Autodesk Inventor part; units mm, degrees
(part 2 of 3)
  line L420 (576.2805, 16.5874) -> (576.1711, 16.519)
  line L421 (576.1711, 16.519) -> (576.0571, 16.4584)
  line L422 (576.0571, 16.4584) -> (575.9392, 16.4059)
  line L423 (575.9392, 16.4059) -> (575.8179, 16.3617)
  line L424 (575.8179, 16.3617) -> (575.6938, 16.3262)
  line L425 (575.6938, 16.3262) -> (575.5676, 16.2993)
  line L426 (575.5676, 16.2993) -> (575.4398, 16.2814)
  line L427 (575.4398, 16.2814) -> (575.311, 16.2724)
  line L428 (575.311, 16.2724) -> (575.182, 16.2724)
  line L429 (575.182, 16.2724) -> (575.0532, 16.2814)
  line L430 (575.0532, 16.2814) -> (574.9254, 16.2993)
  line L431 (574.9254, 16.2993) -> (574.7992, 16.3262)
  line L432 (574.7992, 16.3262) -> (574.6751, 16.3617)
  line L433 (574.6751, 16.3617) -> (574.5538, 16.4059)
  line L434 (574.5538, 16.4059) -> (574.4359, 16.4584)
  line L435 (574.4359, 16.4584) -> (574.3219, 16.519)
  line L436 (574.3219, 16.519) -> (574.2125, 16.5874)
  line L437 (574.2125, 16.5874) -> (574.1081, 16.6632)
  line L438 (574.1081, 16.6632) -> (574.0092, 16.7462)
  line L439 (574.0092, 16.7462) -> (573.9164, 16.8359)
  line L440 (573.9164, 16.8359) -> (573.83, 16.9318)
  line L441 (573.83, 16.9318) -> (573.7505, 17.0335)
  line L442 (573.7505, 17.0335) -> (573.6784, 17.1405)
  line L443 (573.6784, 17.1405) -> (573.6138, 17.2523)
  line L444 (573.6138, 17.2523) -> (573.5572, 17.3683)
  line L445 (573.5572, 17.3683) -> (573.5089, 17.4879)
  line L446 (573.5089, 17.4879) -> (573.469, 17.6107)
  line L447 (573.469, 17.6107) -> (573.4378, 17.7359)
  line L448 (573.4378, 17.7359) -> (573.4154, 17.863)
  line L449 (573.4154, 17.863) -> (573.4019, 17.9914)
  line L450 (573.4019, 17.9914) -> (573.3974, 18.1204)
  line L451 (573.3974, 18.1204) -> (573.4019, 18.2493)
  line L452 (573.4019, 18.2493) -> (573.4154, 18.3777)
  line L453 (573.4154, 18.3777) -> (573.4378, 18.5048)
  line L454 (573.4378, 18.5048) -> (573.469, 18.63)
  line L455 (573.469, 18.63) -> (573.5089, 18.7528)
  line L456 (573.5089, 18.7528) -> (573.5572, 18.8725)
  line L457 (573.5572, 18.8725) -> (573.6138, 18.9885)
  line L458 (573.6138, 18.9885) -> (573.6784, 19.1002)
  line L459 (573.6784, 19.1002) -> (573.7505, 19.2072)
  line L460 (573.7505, 19.2072) -> (573.83, 19.309)
  line L461 (573.83, 19.309) -> (573.9164, 19.4049)
  line L462 (573.9164, 19.4049) -> (574.0092, 19.4945)
  line L463 (574.0092, 19.4945) -> (574.1081, 19.5775)
  line L464 (574.1081, 19.5775) -> (574.2125, 19.6533)
  line L465 (574.2125, 19.6533) -> (574.3219, 19.7217)
  line L466 (574.3219, 19.7217) -> (574.4359, 19.7823)
  line L467 (574.4359, 19.7823) -> (574.5538, 19.8348)
  line L468 (574.5538, 19.8348) -> (574.6751, 19.879)
  line L469 (574.6751, 19.879) -> (574.7992, 19.9146)
  line L470 (574.7992, 19.9146) -> (574.9254, 19.9414)
  line L471 (574.9254, 19.9414) -> (575.0532, 19.9594)
  line L472 (575.0532, 19.9594) -> (575.182, 19.9684)
  line L473 (575.182, 19.9684) -> (575.311, 19.9684)
  line L474 (575.311, 19.9684) -> (575.4398, 19.9594)
  line L475 (575.4398, 19.9594) -> (575.5676, 19.9414)
  line L476 (575.5676, 19.9414) -> (575.6938, 19.9146)
  line L477 (575.6938, 19.9146) -> (575.8179, 19.879)
  line L478 (575.8179, 19.879) -> (575.9392, 19.8348)
  line L479 (575.9392, 19.8348) -> (576.0571, 19.7823)
  line L480 (576.0571, 19.7823) -> (576.1711, 19.7217)
  line L481 (576.1711, 19.7217) -> (576.2805, 19.6533)
  line L482 (576.2805, 19.6533) -> (576.3849, 19.5775)
  line L483 (576.3849, 19.5775) -> (576.4838, 19.4945)
  line L484 (576.4838, 19.4945) -> (576.5766, 19.4049)
  line L485 (576.5766, 19.4049) -> (576.663, 19.309)
  line L486 (576.663, 19.309) -> (576.7425, 19.2072)
  line L487 (576.7425, 19.2072) -> (576.8146, 19.1002)
  line L488 (576.8146, 19.1002) -> (576.8792, 18.9885)
  line L489 (576.8792, 18.9885) -> (576.9358, 18.8725)
  line L490 (576.9358, 18.8725) -> (576.9841, 18.7528)
  line L491 (576.9841, 18.7528) -> (577.024, 18.63)
  line L492 (577.024, 18.63) -> (577.0552, 18.5048)
  line L493 (577.0552, 18.5048) -> (577.0776, 18.3777)
  line L494 (577.0776, 18.3777) -> (577.0911, 18.2493)
  line L495 (577.0911, 18.2493) -> (577.0956, 18.1204)
  line L496 (314.1597, 166.8545) -> (568.1597, 166.8545)
  line L497 (568.1597, 166.8545) -> (568.1597, 104.8556)
  line L498 (568.1597, 104.8556) -> (314.1597, 104.8556)
  line L499 (314.1597, 104.8556) -> (314.1597, 166.8545)
  line L500 (506.5418, 136.7199) -> (506.585, 137.6267)
  line L501 (506.585, 137.6267) -> (506.7146, 138.5208)
  line L502 (506.7146, 138.5208) -> (506.9254, 139.3996)
  line L503 (506.9254, 139.3996) -> (507.2226, 140.2581)
  line L504 (507.2226, 140.2581) -> (507.601, 141.0785)
  line L505 (507.601, 141.0785) -> (508.0506, 141.8634)
  line L506 (508.0506, 141.8634) -> (508.5764, 142.6025)
  line L507 (508.5764, 142.6025) -> (509.1707, 143.2883)
  line L508 (509.1707, 143.2883) -> (509.8261, 143.9132)
  line L509 (509.8261, 143.9132) -> (510.5398, 144.4694)
  line L510 (510.5398, 144.4694) -> (511.3018, 144.9597)
  line L511 (511.3018, 144.9597) -> (512.1044, 145.3762)
  line L512 (512.1044, 145.3762) -> (512.9452, 145.7115)
  line L513 (512.9452, 145.7115) -> (513.8139, 145.9655)
  line L514 (513.8139, 145.9655) -> (514.6978, 146.1382)
  line L515 (514.6978, 146.1382) -> (515.6046, 146.222)
  line L516 (515.6046, 146.222) -> (516.5113, 146.222)
  line L517 (516.5113, 146.222) -> (517.4105, 146.1382)
  line L518 (517.4105, 146.1382) -> (518.2995, 145.9655)
  line L519 (518.2995, 145.9655) -> (519.1682, 145.7115)
  line L520 (519.1682, 145.7115) -> (520.0115, 145.3762)
  line L521 (520.0115, 145.3762) -> (520.8141, 144.9597)
  line L522 (520.8141, 144.9597) -> (521.5761, 144.4694)
  line L523 (521.5761, 144.4694) -> (522.2873, 143.9132)
  line L524 (522.2873, 143.9132) -> (522.9426, 143.2883)
  line L525 (522.9426, 143.2883) -> (523.5344, 142.6025)
  line L526 (523.5344, 142.6025) -> (524.0602, 141.8634)
  line L527 (524.0602, 141.8634) -> (524.5123, 141.0785)
  line L528 (524.5123, 141.0785) -> (524.8908, 140.2581)
  line L529 (524.8908, 140.2581) -> (525.1854, 139.3996)
  line L530 (525.1854, 139.3996) -> (525.4013, 138.5208)
  line L531 (525.4013, 138.5208) -> (525.5258, 137.6267)
  line L532 (525.5258, 137.6267) -> (525.5715, 136.7199)
  line L533 (525.5715, 136.7199) -> (525.5258, 135.8157)
  line L534 (525.5258, 135.8157) -> (525.4013, 134.919)
  line L535 (525.4013, 134.919) -> (525.1854, 134.0427)
  line L536 (525.1854, 134.0427) -> (524.8908, 133.1842)
  line L537 (524.8908, 133.1842) -> (524.5123, 132.3613)
  line L538 (524.5123, 132.3613) -> (524.0602, 131.5764)
  line L539 (524.0602, 131.5764) -> (523.5344, 130.8373)
  line L540 (523.5344, 130.8373) -> (522.9426, 130.154)
  line L541 (522.9426, 130.154) -> (522.2873, 129.5292)
  line L542 (522.2873, 129.5292) -> (521.5761, 128.9678)
  line L543 (521.5761, 128.9678) -> (520.8141, 128.4827)
  line L544 (520.8141, 128.4827) -> (520.0115, 128.0661)
  line L545 (520.0115, 128.0661) -> (519.1682, 127.7308)
  line L546 (519.1682, 127.7308) -> (518.2995, 127.4718)
  line L547 (518.2995, 127.4718) -> (517.4105, 127.3041)
  line L548 (517.4105, 127.3041) -> (516.5113, 127.2152)
  line L549 (516.5113, 127.2152) -> (515.6046, 127.2152)
  line L550 (515.6046, 127.2152) -> (514.6978, 127.3041)
  line L551 (514.6978, 127.3041) -> (513.8139, 127.4718)
  line L552 (513.8139, 127.4718) -> (512.9452, 127.7308)
  line L553 (512.9452, 127.7308) -> (512.1044, 128.0661)
  line L554 (512.1044, 128.0661) -> (511.3018, 128.4827)
  line L555 (511.3018, 128.4827) -> (510.5398, 128.9678)
  line L556 (510.5398, 128.9678) -> (509.8261, 129.5292)
  line L557 (509.8261, 129.5292) -> (509.1707, 130.154)
  line L558 (509.1707, 130.154) -> (508.5764, 130.8373)
  line L559 (508.5764, 130.8373) -> (508.0506, 131.5764)
  line L560 (508.0506, 131.5764) -> (507.601, 132.3613)
  line L561 (507.601, 132.3613) -> (507.2226, 133.1842)
  line L562 (507.2226, 133.1842) -> (506.9254, 134.0427)
  line L563 (506.9254, 134.0427) -> (506.7146, 134.919)
  line L564 (506.7146, 134.919) -> (506.585, 135.8157)
  line L565 (506.585, 135.8157) -> (506.5418, 136.7199)
  line L566 (401.8837, 136.7199) -> (401.9269, 137.6267)
  line L567 (401.9269, 137.6267) -> (402.0564, 138.5208)
  line L568 (402.0564, 138.5208) -> (402.2647, 139.3996)
  line L569 (402.2647, 139.3996) -> (402.5644, 140.2581)
  line L570 (402.5644, 140.2581) -> (402.9429, 141.0785)
  line L571 (402.9429, 141.0785) -> (403.3924, 141.8634)
  line L572 (403.3924, 141.8634) -> (403.9182, 142.6025)
  line L573 (403.9182, 142.6025) -> (404.5126, 143.2883)
  line L574 (404.5126, 143.2883) -> (405.1679, 143.9132)
  line L575 (405.1679, 143.9132) -> (405.8791, 144.4694)
  line L576 (405.8791, 144.4694) -> (406.6411, 144.9597)
  line L577 (406.6411, 144.9597) -> (407.4463, 145.3762)
  line L578 (407.4463, 145.3762) -> (408.287, 145.7115)
  line L579 (408.287, 145.7115) -> (409.1532, 145.9655)
  line L580 (409.1532, 145.9655) -> (410.0422, 146.1382)
  line L581 (410.0422, 146.1382) -> (410.9464, 146.222)
  line L582 (410.9464, 146.222) -> (411.8481, 146.222)
  line L583 (411.8481, 146.222) -> (412.7523, 146.1382)
  line L584 (412.7523, 146.1382) -> (413.6413, 145.9655)
  line L585 (413.6413, 145.9655) -> (414.51, 145.7115)
  line L586 (414.51, 145.7115) -> (415.3533, 145.3762)
  line L587 (415.3533, 145.3762) -> (416.1534, 144.9597)
  line L588 (416.1534, 144.9597) -> (416.9179, 144.4694)
  line L589 (416.9179, 144.4694) -> (417.6266, 143.9132)
  line L590 (417.6266, 143.9132) -> (418.2845, 143.2883)
  line L591 (418.2845, 143.2883) -> (418.8763, 142.6025)
  line L592 (418.8763, 142.6025) -> (419.4021, 141.8634)
  line L593 (419.4021, 141.8634) -> (419.8542, 141.0785)
  line L594 (419.8542, 141.0785) -> (420.2301, 140.2581)
  line L595 (420.2301, 140.2581) -> (420.5273, 139.3996)
  line L596 (420.5273, 139.3996) -> (420.7381, 138.5208)
  line L597 (420.7381, 138.5208) -> (420.8702, 137.6267)
  line L598 (420.8702, 137.6267) -> (420.9108, 136.7199)
  line L599 (420.9108, 136.7199) -> (420.8702, 135.8157)
  line L600 (420.8702, 135.8157) -> (420.7381, 134.919)
  line L601 (420.7381, 134.919) -> (420.5273, 134.0427)
  line L602 (420.5273, 134.0427) -> (420.2301, 133.1842)
  line L603 (420.2301, 133.1842) -> (419.8542, 132.3613)
  line L604 (419.8542, 132.3613) -> (419.4021, 131.5764)
  line L605 (419.4021, 131.5764) -> (418.8763, 130.8373)
  line L606 (418.8763, 130.8373) -> (418.2845, 130.154)
  line L607 (418.2845, 130.154) -> (417.6266, 129.5292)
  line L608 (417.6266, 129.5292) -> (416.9179, 128.9678)
  line L609 (416.9179, 128.9678) -> (416.1534, 128.4827)
  line L610 (416.1534, 128.4827) -> (415.3533, 128.0661)
  line L611 (415.3533, 128.0661) -> (414.51, 127.7308)
  line L612 (414.51, 127.7308) -> (413.6413, 127.4718)
  line L613 (413.6413, 127.4718) -> (412.7523, 127.3041)
  line L614 (412.7523, 127.3041) -> (411.8481, 127.2152)
  line L615 (411.8481, 127.2152) -> (410.9464, 127.2152)
  line L616 (410.9464, 127.2152) -> (410.0422, 127.3041)
  line L617 (410.0422, 127.3041) -> (409.1532, 127.4718)
  line L618 (409.1532, 127.4718) -> (408.287, 127.7308)
  line L619 (408.287, 127.7308) -> (407.4463, 128.0661)
  line L620 (407.4463, 128.0661) -> (406.6411, 128.4827)
  line L621 (406.6411, 128.4827) -> (405.8791, 128.9678)
  line L622 (405.8791, 128.9678) -> (405.1679, 129.5292)
  line L623 (405.1679, 129.5292) -> (404.5126, 130.154)
  line L624 (404.5126, 130.154) -> (403.9182, 130.8373)
  line L625 (403.9182, 130.8373) -> (403.3924, 131.5764)
  line L626 (403.3924, 131.5764) -> (402.9429, 132.3613)
  line L627 (402.9429, 132.3613) -> (402.5644, 133.1842)
  line L628 (402.5644, 133.1842) -> (402.2647, 134.0427)
  line L629 (402.2647, 134.0427) -> (402.0564, 134.919)
  line L630 (402.0564, 134.919) -> (401.9269, 135.8157)
  line L631 (401.9269, 135.8157) -> (401.8837, 136.7199)
  line L632 (340.0423, 136.7199) -> (340.0829, 137.6267)
  line L633 (340.0829, 137.6267) -> (340.2099, 138.5208)
  line L634 (340.2099, 138.5208) -> (340.4258, 139.3996)
  line L635 (340.4258, 139.3996) -> (340.723, 140.2581)
  line L636 (340.723, 140.2581) -> (341.0964, 141.0785)
  line L637 (341.0964, 141.0785) -> (341.5511, 141.8634)
  line L638 (341.5511, 141.8634) -> (342.0768, 142.6025)
  line L639 (342.0768, 142.6025) -> (342.6687, 143.2883)
  line L640 (342.6687, 143.2883) -> (343.3214, 143.9132)
  line L641 (343.3214, 143.9132) -> (344.0352, 144.4694)
  line L642 (344.0352, 144.4694) -> (344.7972, 144.9597)
  line L643 (344.7972, 144.9597) -> (345.5998, 145.3762)
  line L644 (345.5998, 145.3762) -> (346.4406, 145.7115)
  line L645 (346.4406, 145.7115) -> (347.3118, 145.9655)
  line L646 (347.3118, 145.9655) -> (348.2008, 146.1382)
  line L647 (348.2008, 146.1382) -> (349.0999, 146.222)
  line L648 (349.0999, 146.222) -> (350.0067, 146.222)
  line L649 (350.0067, 146.222) -> (350.9059, 146.1382)
  line L650 (350.9059, 146.1382) -> (351.7949, 145.9655)
  line L651 (351.7949, 145.9655) -> (352.6661, 145.7115)
  line L652 (352.6661, 145.7115) -> (353.5068, 145.3762)
  line L653 (353.5068, 145.3762) -> (354.312, 144.9597)
  line L654 (354.312, 144.9597) -> (355.074, 144.4694)
  line L655 (355.074, 144.4694) -> (355.7852, 143.9132)
  line L656 (355.7852, 143.9132) -> (356.438, 143.2883)
  line L657 (356.438, 143.2883) -> (357.0349, 142.6025)
  line L658 (357.0349, 142.6025) -> (357.5556, 141.8634)
  line L659 (357.5556, 141.8634) -> (358.0128, 141.0785)
  line L660 (358.0128, 141.0785) -> (358.3862, 140.2581)
  line L661 (358.3862, 140.2581) -> (358.6834, 139.3996)
  line L662 (358.6834, 139.3996) -> (358.8942, 138.5208)
  line L663 (358.8942, 138.5208) -> (359.0212, 137.6267)
  line L664 (359.0212, 137.6267) -> (359.0694, 136.7199)
  line L665 (359.0694, 136.7199) -> (359.0212, 135.8157)
  line L666 (359.0212, 135.8157) -> (358.8942, 134.919)
  line L667 (358.8942, 134.919) -> (358.6834, 134.0427)
  line L668 (358.6834, 134.0427) -> (358.3862, 133.1842)
  line L669 (358.3862, 133.1842) -> (358.0128, 132.3613)
  line L670 (358.0128, 132.3613) -> (357.5556, 131.5764)
  line L671 (357.5556, 131.5764) -> (357.0349, 130.8373)
  line L672 (357.0349, 130.8373) -> (356.438, 130.154)
  line L673 (356.438, 130.154) -> (355.7852, 129.5292)
  line L674 (355.7852, 129.5292) -> (355.074, 128.9678)
  line L675 (355.074, 128.9678) -> (354.312, 128.4827)
  line L676 (354.312, 128.4827) -> (353.5068, 128.0661)
  line L677 (353.5068, 128.0661) -> (352.6661, 127.7308)
  line L678 (352.6661, 127.7308) -> (351.7949, 127.4718)
  line L679 (351.7949, 127.4718) -> (350.9059, 127.3041)
  line L680 (350.9059, 127.3041) -> (350.0067, 127.2152)
  line L681 (350.0067, 127.2152) -> (349.0999, 127.2152)
  line L682 (349.0999, 127.2152) -> (348.2008, 127.3041)
  line L683 (348.2008, 127.3041) -> (347.3118, 127.4718)
  line L684 (347.3118, 127.4718) -> (346.4406, 127.7308)
  line L685 (346.4406, 127.7308) -> (345.5998, 128.0661)
  line L686 (345.5998, 128.0661) -> (344.7972, 128.4827)
  line L687 (344.7972, 128.4827) -> (344.0352, 128.9678)
  line L688 (344.0352, 128.9678) -> (343.3214, 129.5292)
  line L689 (343.3214, 129.5292) -> (342.6687, 130.154)
  line L690 (342.6687, 130.154) -> (342.0768, 130.8373)
  line L691 (342.0768, 130.8373) -> (341.5511, 131.5764)
  line L692 (341.5511, 131.5764) -> (341.0964, 132.3613)
  line L693 (341.0964, 132.3613) -> (340.723, 133.1842)
  line L694 (340.723, 133.1842) -> (340.4258, 134.0427)
  line L695 (340.4258, 134.0427) -> (340.2099, 134.919)
  line L696 (340.2099, 134.919) -> (340.0829, 135.8157)
  line L697 (340.0829, 135.8157) -> (340.0423, 136.7199)
  line L698 (319.4988, 163.174) -> (319.4943, 163.045)
  line L699 (319.4943, 163.045) -> (319.4808, 162.9167)
  line L700 (319.4808, 162.9167) -> (319.4584, 162.7895)
  line L701 (319.4584, 162.7895) -> (319.4271, 162.6643)
  line L702 (319.4271, 162.6643) -> (319.3873, 162.5416)
  line L703 (319.3873, 162.5416) -> (319.3389, 162.4219)
  line L704 (319.3389, 162.4219) -> (319.2823, 162.3059)
  line L705 (319.2823, 162.3059) -> (319.2178, 162.1941)
  line L706 (319.2178, 162.1941) -> (319.1456, 162.0871)
  line L707 (319.1456, 162.0871) -> (319.0662, 161.9854)
  line L708 (319.0662, 161.9854) -> (318.9798, 161.8895)
  line L709 (318.9798, 161.8895) -> (318.887, 161.7998)
  line L710 (318.887, 161.7998) -> (318.7881, 161.7169)
  line L711 (318.7881, 161.7169) -> (318.6837, 161.641)
  line L712 (318.6837, 161.641) -> (318.5742, 161.5726)
  line L713 (318.5742, 161.5726) -> (318.4603, 161.512)
  line L714 (318.4603, 161.512) -> (318.3424, 161.4595)
  line L715 (318.3424, 161.4595) -> (318.2211, 161.4154)
  line L716 (318.2211, 161.4154) -> (318.097, 161.3798)
  line L717 (318.097, 161.3798) -> (317.9708, 161.353)
  line L718 (317.9708, 161.353) -> (317.8429, 161.335)
  line L719 (317.8429, 161.335) -> (317.7142, 161.326)
  line L720 (317.7142, 161.326) -> (317.5851, 161.326)
  line L721 (317.5851, 161.326) -> (317.4564, 161.335)
  line L722 (317.4564, 161.335) -> (317.3286, 161.353)
  line L723 (317.3286, 161.353) -> (317.2023, 161.3798)
  line L724 (317.2023, 161.3798) -> (317.0783, 161.4154)
  line L725 (317.0783, 161.4154) -> (316.957, 161.4595)
  line L726 (316.957, 161.4595) -> (316.8391, 161.512)
  line L727 (316.8391, 161.512) -> (316.7251, 161.5726)
  line L728 (316.7251, 161.5726) -> (316.6156, 161.641)
  line L729 (316.6156, 161.641) -> (316.5112, 161.7169)
  line L730 (316.5112, 161.7169) -> (316.4124, 161.7998)
  line L731 (316.4124, 161.7998) -> (316.3195, 161.8895)
  line L732 (316.3195, 161.8895) -> (316.2332, 161.9854)
  line L733 (316.2332, 161.9854) -> (316.1537, 162.0871)
  line L734 (316.1537, 162.0871) -> (316.0815, 162.1941)
  line L735 (316.0815, 162.1941) -> (316.017, 162.3059)
  line L736 (316.017, 162.3059) -> (315.9604, 162.4219)
  line L737 (315.9604, 162.4219) -> (315.9121, 162.5416)
  line L738 (315.9121, 162.5416) -> (315.8722, 162.6643)
  line L739 (315.8722, 162.6643) -> (315.8409, 162.7895)
  line L740 (315.8409, 162.7895) -> (315.8185, 162.9167)
  line L741 (315.8185, 162.9167) -> (315.805, 163.045)
  line L742 (315.805, 163.045) -> (315.8005, 163.174)
  line L743 (315.8005, 163.174) -> (315.805, 163.303)
  line L744 (315.805, 163.303) -> (315.8185, 163.4313)
  line L745 (315.8185, 163.4313) -> (315.8409, 163.5585)
  line L746 (315.8409, 163.5585) -> (315.8722, 163.6837)
  line L747 (315.8722, 163.6837) -> (315.9121, 163.8064)
  line L748 (315.9121, 163.8064) -> (315.9604, 163.9261)
  line L749 (315.9604, 163.9261) -> (316.017, 164.0421)
  line L750 (316.017, 164.0421) -> (316.0815, 164.1539)
  line L751 (316.0815, 164.1539) -> (316.1537, 164.2609)
  line L752 (316.1537, 164.2609) -> (316.2332, 164.3626)
  line L753 (316.2332, 164.3626) -> (316.3195, 164.4585)
  line L754 (316.3195, 164.4585) -> (316.4124, 164.5482)
  line L755 (316.4124, 164.5482) -> (316.5112, 164.6311)
  line L756 (316.5112, 164.6311) -> (316.6156, 164.707)
  line L757 (316.6156, 164.707) -> (316.7251, 164.7754)
  line L758 (316.7251, 164.7754) -> (316.8391, 164.836)
  line L759 (316.8391, 164.836) -> (316.957, 164.8885)
  line L760 (316.957, 164.8885) -> (317.0783, 164.9326)
  line L761 (317.0783, 164.9326) -> (317.2023, 164.9682)
  line L762 (317.2023, 164.9682) -> (317.3286, 164.995)
  line L763 (317.3286, 164.995) -> (317.4564, 165.013)
  line L764 (317.4564, 165.013) -> (317.5851, 165.022)
  line L765 (317.5851, 165.022) -> (317.7142, 165.022)
  line L766 (317.7142, 165.022) -> (317.8429, 165.013)
  line L767 (317.8429, 165.013) -> (317.9708, 164.995)
  line L768 (317.9708, 164.995) -> (318.097, 164.9682)
  line L769 (318.097, 164.9682) -> (318.2211, 164.9326)
  line L770 (318.2211, 164.9326) -> (318.3424, 164.8885)
  line L771 (318.3424, 164.8885) -> (318.4603, 164.836)
  line L772 (318.4603, 164.836) -> (318.5742, 164.7754)
  line L773 (318.5742, 164.7754) -> (318.6837, 164.707)
  line L774 (318.6837, 164.707) -> (318.7881, 164.6311)
  line L775 (318.7881, 164.6311) -> (318.887, 164.5482)
  line L776 (318.887, 164.5482) -> (318.9798, 164.4585)
  line L777 (318.9798, 164.4585) -> (319.0662, 164.3626)
  line L778 (319.0662, 164.3626) -> (319.1456, 164.2609)
  line L779 (319.1456, 164.2609) -> (319.2178, 164.1539)
  line L780 (319.2178, 164.1539) -> (319.2823, 164.0421)
  line L781 (319.2823, 164.0421) -> (319.3389, 163.9261)
  line L782 (319.3389, 163.9261) -> (319.3873, 163.8064)
  line L783 (319.3873, 163.8064) -> (319.4271, 163.6837)
  line L784 (319.4271, 163.6837) -> (319.4584, 163.5585)
  line L785 (319.4584, 163.5585) -> (319.4808, 163.4313)
  line L786 (319.4808, 163.4313) -> (319.4943, 163.303)
  line L787 (319.4943, 163.303) -> (319.4988, 163.174)
  line L788 (319.4988, 108.9831) -> (319.4943, 108.8541)
  line L789 (319.4943, 108.8541) -> (319.4808, 108.7258)
  line L790 (319.4808, 108.7258) -> (319.4584, 108.5986)
  line L791 (319.4584, 108.5986) -> (319.4271, 108.4734)
  line L792 (319.4271, 108.4734) -> (319.3873, 108.3507)
  line L793 (319.3873, 108.3507) -> (319.3389, 108.231)
  line L794 (319.3389, 108.231) -> (319.2823, 108.115)
  line L795 (319.2823, 108.115) -> (319.2178, 108.0032)
  line L796 (319.2178, 108.0032) -> (319.1456, 107.8962)
  line L797 (319.1456, 107.8962) -> (319.0662, 107.7945)
  line L798 (319.0662, 107.7945) -> (318.9798, 107.6986)
  line L799 (318.9798, 107.6986) -> (318.887, 107.6089)
  line L800 (318.887, 107.6089) -> (318.7881, 107.526)
  line L801 (318.7881, 107.526) -> (318.6837, 107.4501)
  line L802 (318.6837, 107.4501) -> (318.5742, 107.3817)
  line L803 (318.5742, 107.3817) -> (318.4603, 107.3211)
  line L804 (318.4603, 107.3211) -> (318.3424, 107.2686)
  line L805 (318.3424, 107.2686) -> (318.2211, 107.2245)
  line L806 (318.2211, 107.2245) -> (318.097, 107.1889)
  line L807 (318.097, 107.1889) -> (317.9708, 107.1621)
  line L808 (317.9708, 107.1621) -> (317.8429, 107.1441)
  line L809 (317.8429, 107.1441) -> (317.7142, 107.1351)
  line L810 (317.7142, 107.1351) -> (317.5851, 107.1351)
  line L811 (317.5851, 107.1351) -> (317.4564, 107.1441)
  line L812 (317.4564, 107.1441) -> (317.3286, 107.1621)
  line L813 (317.3286, 107.1621) -> (317.2023, 107.1889)
  line L814 (317.2023, 107.1889) -> (317.0783, 107.2245)
  line L815 (317.0783, 107.2245) -> (316.957, 107.2686)
  line L816 (316.957, 107.2686) -> (316.8391, 107.3211)
  line L817 (316.8391, 107.3211) -> (316.7251, 107.3817)
  line L818 (316.7251, 107.3817) -> (316.6156, 107.4501)
  line L819 (316.6156, 107.4501) -> (316.5112, 107.526)
  line L820 (316.5112, 107.526) -> (316.4124, 107.6089)
  line L821 (316.4124, 107.6089) -> (316.3195, 107.6986)
  line L822 (316.3195, 107.6986) -> (316.2332, 107.7945)
  line L823 (316.2332, 107.7945) -> (316.1537, 107.8962)
  line L824 (316.1537, 107.8962) -> (316.0815, 108.0032)
  line L825 (316.0815, 108.0032) -> (316.017, 108.115)
  line L826 (316.017, 108.115) -> (315.9604, 108.231)
  line L827 (315.9604, 108.231) -> (315.9121, 108.3507)
  line L828 (315.9121, 108.3507) -> (315.8722, 108.4734)
  line L829 (315.8722, 108.4734) -> (315.8409, 108.5986)
  line L830 (315.8409, 108.5986) -> (315.8185, 108.7258)
  line L831 (315.8185, 108.7258) -> (315.805, 108.8541)
  line L832 (315.805, 108.8541) -> (315.8005, 108.9831)
  line L833 (315.8005, 108.9831) -> (315.805, 109.1121)
  line L834 (315.805, 109.1121) -> (315.8185, 109.2404)
  line L835 (315.8185, 109.2404) -> (315.8409, 109.3676)
  line L836 (315.8409, 109.3676) -> (315.8722, 109.4928)
  line L837 (315.8722, 109.4928) -> (315.9121, 109.6155)
  line L838 (315.9121, 109.6155) -> (315.9604, 109.7352)
  line L839 (315.9604, 109.7352) -> (316.017, 109.8512)
  line L840 (316.017, 109.8512) -> (316.0815, 109.963)
  line L841 (316.0815, 109.963) -> (316.1537, 110.07)
  line L842 (316.1537, 110.07) -> (316.2332, 110.1717)
  line L843 (316.2332, 110.1717) -> (316.3195, 110.2676)
  line L844 (316.3195, 110.2676) -> (316.4124, 110.3573)
  line L845 (316.4124, 110.3573) -> (316.5112, 110.4402)
  line L846 (316.5112, 110.4402) -> (316.6156, 110.5161)
  line L847 (316.6156, 110.5161) -> (316.7251, 110.5845)
  line L848 (316.7251, 110.5845) -> (316.8391, 110.6451)
  line L849 (316.8391, 110.6451) -> (316.957, 110.6976)
  line L850 (316.957, 110.6976) -> (317.0783, 110.7417)
  line L851 (317.0783, 110.7417) -> (317.2023, 110.7773)
  line L852 (317.2023, 110.7773) -> (317.3286, 110.8041)
  line L853 (317.3286, 110.8041) -> (317.4564, 110.8221)
  line L854 (317.4564, 110.8221) -> (317.5851, 110.8311)
  line L855 (317.5851, 110.8311) -> (317.7142, 110.8311)
  line L856 (317.7142, 110.8311) -> (317.8429, 110.8221)
  line L857 (317.8429, 110.8221) -> (317.9708, 110.8041)
  line L858 (317.9708, 110.8041) -> (318.097, 110.7773)
  line L859 (318.097, 110.7773) -> (318.2211, 110.7417)
  line L860 (318.2211, 110.7417) -> (318.3424, 110.6976)
  line L861 (318.3424, 110.6976) -> (318.4603, 110.6451)
  line L862 (318.4603, 110.6451) -> (318.5742, 110.5845)
  line L863 (318.5742, 110.5845) -> (318.6837, 110.5161)
  line L864 (318.6837, 110.5161) -> (318.7881, 110.4402)
  line L865 (318.7881, 110.4402) -> (318.887, 110.3573)
  line L866 (318.887, 110.3573) -> (318.9798, 110.2676)
  line L867 (318.9798, 110.2676) -> (319.0662, 110.1717)
  line L868 (319.0662, 110.1717) -> (319.1456, 110.07)
  line L869 (319.1456, 110.07) -> (319.2178, 109.963)
  line L870 (319.2178, 109.963) -> (319.2823, 109.8512)
  line L871 (319.2823, 109.8512) -> (319.3389, 109.7352)
  line L872 (319.3389, 109.7352) -> (319.3873, 109.6155)
  line L873 (319.3873, 109.6155) -> (319.4271, 109.4928)
  line L874 (319.4271, 109.4928) -> (319.4584, 109.3676)
  line L875 (319.4584, 109.3676) -> (319.4808, 109.2404)
  line L876 (319.4808, 109.2404) -> (319.4943, 109.1121)
  line L877 (319.4943, 109.1121) -> (319.4988, 108.9831)
  line L878 (565.8483, 108.9831) -> (565.8438, 108.8541)
  line L879 (565.8438, 108.8541) -> (565.8303, 108.7258)
  line L880 (565.8303, 108.7258) -> (565.8079, 108.5986)
  line L881 (565.8079, 108.5986) -> (565.7767, 108.4734)
  line L882 (565.7767, 108.4734) -> (565.7368, 108.3507)
  line L883 (565.7368, 108.3507) -> (565.6884, 108.231)
  line L884 (565.6884, 108.231) -> (565.6319, 108.115)
  line L885 (565.6319, 108.115) -> (565.5673, 108.0032)
  line L886 (565.5673, 108.0032) -> (565.4951, 107.8962)
  line L887 (565.4951, 107.8962) -> (565.4157, 107.7945)
  line L888 (565.4157, 107.7945) -> (565.3293, 107.6986)
  line L889 (565.3293, 107.6986) -> (565.2365, 107.6089)
  line L890 (565.2365, 107.6089) -> (565.1376, 107.526)
  line L891 (565.1376, 107.526) -> (565.0332, 107.4501)
  line L892 (565.0332, 107.4501) -> (564.9237, 107.3817)
  line L893 (564.9237, 107.3817) -> (564.8098, 107.3211)
  line L894 (564.8098, 107.3211) -> (564.6919, 107.2686)
  line L895 (564.6919, 107.2686) -> (564.5706, 107.2245)
  line L896 (564.5706, 107.2245) -> (564.4465, 107.1889)
  line L897 (564.4465, 107.1889) -> (564.3203, 107.1621)
  line L898 (564.3203, 107.1621) -> (564.1925, 107.1441)
  line L899 (564.1925, 107.1441) -> (564.0637, 107.1351)
  line L900 (564.0637, 107.1351) -> (563.9346, 107.1351)
  line L901 (563.9346, 107.1351) -> (563.8059, 107.1441)
  line L902 (563.8059, 107.1441) -> (563.6781, 107.1621)
  line L903 (563.6781, 107.1621) -> (563.5518, 107.1889)
  line L904 (563.5518, 107.1889) -> (563.4278, 107.2245)
  line L905 (563.4278, 107.2245) -> (563.3065, 107.2686)
  line L906 (563.3065, 107.2686) -> (563.1886, 107.3211)
  line L907 (563.1886, 107.3211) -> (563.0746, 107.3817)
  line L908 (563.0746, 107.3817) -> (562.9652, 107.4501)
  line L909 (562.9652, 107.4501) -> (562.8607, 107.526)
  line L910 (562.8607, 107.526) -> (562.7619, 107.6089)
  line L911 (562.7619, 107.6089) -> (562.669, 107.6986)
  line L912 (562.669, 107.6986) -> (562.5827, 107.7945)
  line L913 (562.5827, 107.7945) -> (562.5032, 107.8962)
  line L914 (562.5032, 107.8962) -> (562.431, 108.0032)
  line L915 (562.431, 108.0032) -> (562.3665, 108.115)
  line L916 (562.3665, 108.115) -> (562.3099, 108.231)
  line L917 (562.3099, 108.231) -> (562.2616, 108.3507)
  line L918 (562.2616, 108.3507) -> (562.2217, 108.4734)
  line L919 (562.2217, 108.4734) -> (562.1905, 108.5986)
  line L920 (562.1905, 108.5986) -> (562.1681, 108.7258)
  line L921 (562.1681, 108.7258) -> (562.1546, 108.8541)
  line L922 (562.1546, 108.8541) -> (562.1501, 108.9831)
  line L923 (562.1501, 108.9831) -> (562.1546, 109.1121)
  line L924 (562.1546, 109.1121) -> (562.1681, 109.2404)
  line L925 (562.1681, 109.2404) -> (562.1905, 109.3676)
  line L926 (562.1905, 109.3676) -> (562.2217, 109.4928)
  line L927 (562.2217, 109.4928) -> (562.2616, 109.6155)
  line L928 (562.2616, 109.6155) -> (562.3099, 109.7352)
  line L929 (562.3099, 109.7352) -> (562.3665, 109.8512)
  line L930 (562.3665, 109.8512) -> (562.431, 109.963)
  line L931 (562.431, 109.963) -> (562.5032, 110.07)
  line L932 (562.5032, 110.07) -> (562.5827, 110.1717)
  line L933 (562.5827, 110.1717) -> (562.669, 110.2676)
  line L934 (562.669, 110.2676) -> (562.7619, 110.3573)
  line L935 (562.7619, 110.3573) -> (562.8607, 110.4402)
  line L936 (562.8607, 110.4402) -> (562.9652, 110.5161)
  line L937 (562.9652, 110.5161) -> (563.0746, 110.5845)
  line L938 (563.0746, 110.5845) -> (563.1886, 110.6451)
  line L939 (563.1886, 110.6451) -> (563.3065, 110.6976)
  line L940 (563.3065, 110.6976) -> (563.4278, 110.7417)
  line L941 (563.4278, 110.7417) -> (563.5518, 110.7773)
  line L942 (563.5518, 110.7773) -> (563.6781, 110.8041)
  line L943 (563.6781, 110.8041) -> (563.8059, 110.8221)
  line L944 (563.8059, 110.8221) -> (563.9346, 110.8311)
  line L945 (563.9346, 110.8311) -> (564.0637, 110.8311)
  line L946 (564.0637, 110.8311) -> (564.1925, 110.8221)
  line L947 (564.1925, 110.8221) -> (564.3203, 110.8041)
  line L948 (564.3203, 110.8041) -> (564.4465, 110.7773)
  line L949 (564.4465, 110.7773) -> (564.5706, 110.7417)
  line L950 (564.5706, 110.7417) -> (564.6919, 110.6976)
  line L951 (564.6919, 110.6976) -> (564.8098, 110.6451)
  line L952 (564.8098, 110.6451) -> (564.9237, 110.5845)
  line L953 (564.9237, 110.5845) -> (565.0332, 110.5161)
  line L954 (565.0332, 110.5161) -> (565.1376, 110.4402)
  line L955 (565.1376, 110.4402) -> (565.2365, 110.3573)
  line L956 (565.2365, 110.3573) -> (565.3293, 110.2676)
  line L957 (565.3293, 110.2676) -> (565.4157, 110.1717)
  line L958 (565.4157, 110.1717) -> (565.4951, 110.07)
  line L959 (565.4951, 110.07) -> (565.5673, 109.963)
  line L960 (565.5673, 109.963) -> (565.6319, 109.8512)
  line L961 (565.6319, 109.8512) -> (565.6884, 109.7352)
  line L962 (565.6884, 109.7352) -> (565.7368, 109.6155)
  line L963 (565.7368, 109.6155) -> (565.7767, 109.4928)
  line L964 (565.7767, 109.4928) -> (565.8079, 109.3676)
  line L965 (565.8079, 109.3676) -> (565.8303, 109.2404)
  line L966 (565.8303, 109.2404) -> (565.8438, 109.1121)
  line L967 (565.8438, 109.1121) -> (565.8483, 108.9831)
  line L968 (565.8483, 163.174) -> (565.8438, 163.045)
  line L969 (565.8438, 163.045) -> (565.8303, 162.9167)
  line L970 (565.8303, 162.9167) -> (565.8079, 162.7895)
  line L971 (565.8079, 162.7895) -> (565.7767, 162.6643)
  line L972 (565.7767, 162.6643) -> (565.7368, 162.5416)
  line L973 (565.7368, 162.5416) -> (565.6884, 162.4219)
  line L974 (565.6884, 162.4219) -> (565.6319, 162.3059)
  line L975 (565.6319, 162.3059) -> (565.5673, 162.1941)
  line L976 (565.5673, 162.1941) -> (565.4951, 162.0871)
  line L977 (565.4951, 162.0871) -> (565.4157, 161.9854)
  line L978 (565.4157, 161.9854) -> (565.3293, 161.8895)
  line L979 (565.3293, 161.8895) -> (565.2365, 161.7998)
  line L980 (565.2365, 161.7998) -> (565.1376, 161.7169)
  line L981 (565.1376, 161.7169) -> (565.0332, 161.641)
  line L982 (565.0332, 161.641) -> (564.9237, 161.5726)
  line L983 (564.9237, 161.5726) -> (564.8098, 161.512)
  line L984 (564.8098, 161.512) -> (564.6919, 161.4595)
  line L985 (564.6919, 161.4595) -> (564.5706, 161.4154)
  line L986 (564.5706, 161.4154) -> (564.4465, 161.3798)
  line L987 (564.4465, 161.3798) -> (564.3203, 161.353)
  line L988 (564.3203, 161.353) -> (564.1925, 161.335)
  line L989 (564.1925, 161.335) -> (564.0637, 161.326)
  line L990 (564.0637, 161.326) -> (563.9346, 161.326)
  line L991 (563.9346, 161.326) -> (563.8059, 161.335)
  line L992 (563.8059, 161.335) -> (563.6781, 161.353)
  line L993 (563.6781, 161.353) -> (563.5518, 161.3798)
  line L994 (563.5518, 161.3798) -> (563.4278, 161.4154)
  line L995 (563.4278, 161.4154) -> (563.3065, 161.4595)
  line L996 (563.3065, 161.4595) -> (563.1886, 161.512)
  line L997 (563.1886, 161.512) -> (563.0746, 161.5726)
  line L998 (563.0746, 161.5726) -> (562.9652, 161.641)
  line L999 (562.9652, 161.641) -> (562.8607, 161.7169)
  line L1000 (562.8607, 161.7169) -> (562.7619, 161.7998)
  line L1001 (562.7619, 161.7998) -> (562.669, 161.8895)
  line L1002 (562.669, 161.8895) -> (562.5827, 161.9854)
  line L1003 (562.5827, 161.9854) -> (562.5032, 162.0871)
  line L1004 (562.5032, 162.0871) -> (562.431, 162.1941)
  line L1005 (562.431, 162.1941) -> (562.3665, 162.3059)
  line L1006 (562.3665, 162.3059) -> (562.3099, 162.4219)
  line L1007 (562.3099, 162.4219) -> (562.2616, 162.5416)
  line L1008 (562.2616, 162.5416) -> (562.2217, 162.6643)
  line L1009 (562.2217, 162.6643) -> (562.1905, 162.7895)
  line L1010 (562.1905, 162.7895) -> (562.1681, 162.9167)
  line L1011 (562.1681, 162.9167) -> (562.1546, 163.045)
  line L1012 (562.1546, 163.045) -> (562.1501, 163.174)
  line L1013 (562.1501, 163.174) -> (562.1546, 163.303)
  line L1014 (562.1546, 163.303) -> (562.1681, 163.4313)
  line L1015 (562.1681, 163.4313) -> (562.1905, 163.5585)
  line L1016 (562.1905, 163.5585) -> (562.2217, 163.6837)
  line L1017 (562.2217, 163.6837) -> (562.2616, 163.8064)
  line L1018 (562.2616, 163.8064) -> (562.3099, 163.9261)
  line L1019 (562.3099, 163.9261) -> (562.3665, 164.0421)
  line L1020 (562.3665, 164.0421) -> (562.431, 164.1539)
  line L1021 (562.431, 164.1539) -> (562.5032, 164.2609)
  line L1022 (562.5032, 164.2609) -> (562.5827, 164.3626)
  line L1023 (562.5827, 164.3626) -> (562.669, 164.4585)
  line L1024 (562.669, 164.4585) -> (562.7619, 164.5482)
  line L1025 (562.7619, 164.5482) -> (562.8607, 164.6311)
  line L1026 (562.8607, 164.6311) -> (562.9652, 164.707)
  line L1027 (562.9652, 164.707) -> (563.0746, 164.7754)
  line L1028 (563.0746, 164.7754) -> (563.1886, 164.836)
  line L1029 (563.1886, 164.836) -> (563.3065, 164.8885)
  line L1030 (563.3065, 164.8885) -> (563.4278, 164.9326)
  line L1031 (563.4278, 164.9326) -> (563.5518, 164.9682)
  line L1032 (563.5518, 164.9682) -> (563.6781, 164.995)
  line L1033 (563.6781, 164.995) -> (563.8059, 165.013)
  line L1034 (563.8059, 165.013) -> (563.9346, 165.022)
  line L1035 (563.9346, 165.022) -> (564.0637, 165.022)
  line L1036 (564.0637, 165.022) -> (564.1925, 165.013)
  line L1037 (564.1925, 165.013) -> (564.3203, 164.995)
  line L1038 (564.3203, 164.995) -> (564.4465, 164.9682)
  line L1039 (564.4465, 164.9682) -> (564.5706, 164.9326)
  line L1040 (564.5706, 164.9326) -> (564.6919, 164.8885)
  line L1041 (564.6919, 164.8885) -> (564.8098, 164.836)
  line L1042 (564.8098, 164.836) -> (564.9237, 164.7754)
  line L1043 (564.9237, 164.7754) -> (565.0332, 164.707)
  line L1044 (565.0332, 164.707) -> (565.1376, 164.6311)
  line L1045 (565.1376, 164.6311) -> (565.2365, 164.5482)
  line L1046 (565.2365, 164.5482) -> (565.3293, 164.4585)
  line L1047 (565.3293, 164.4585) -> (565.4157, 164.3626)
  line L1048 (565.4157, 164.3626) -> (565.4951, 164.2609)
  line L1049 (565.4951, 164.2609) -> (565.5673, 164.1539)
  line L1050 (565.5673, 164.1539) -> (565.6319, 164.0421)
  line L1051 (565.6319, 164.0421) -> (565.6884, 163.9261)
  line L1052 (565.6884, 163.9261) -> (565.7368, 163.8064)
  line L1053 (565.7368, 163.8064) -> (565.7767, 163.6837)
  line L1054 (565.7767, 163.6837) -> (565.8079, 163.5585)
  line L1055 (565.8079, 163.5585) -> (565.8303, 163.4313)
  line L1056 (565.8303, 163.4313) -> (565.8438, 163.303)
  line L1057 (565.8438, 163.303) -> (565.8483, 163.174)
  line L1058 (419.7983, 121.6831) -> (419.7938, 121.5541)
  line L1059 (419.7938, 121.5541) -> (419.7803, 121.4258)
  line L1060 (419.7803, 121.4258) -> (419.7579, 121.2986)
  line L1061 (419.7579, 121.2986) -> (419.7267, 121.1734)
  line L1062 (419.7267, 121.1734) -> (419.6868, 121.0507)
  line L1063 (419.6868, 121.0507) -> (419.6384, 120.931)
  line L1064 (419.6384, 120.931) -> (419.5819, 120.815)
  line L1065 (419.5819, 120.815) -> (419.5173, 120.7032)
  line L1066 (419.5173, 120.7032) -> (419.4451, 120.5962)
  line L1067 (419.4451, 120.5962) -> (419.3657, 120.4945)
  line L1068 (419.3657, 120.4945) -> (419.2793, 120.3986)
  line L1069 (419.2793, 120.3986) -> (419.1865, 120.3089)
  line L1070 (419.1865, 120.3089) -> (419.0876, 120.226)
  line L1071 (419.0876, 120.226) -> (418.9832, 120.1501)
  line L1072 (418.9832, 120.1501) -> (418.8737, 120.0817)
  line L1073 (418.8737, 120.0817) -> (418.7598, 120.0211)
  line L1074 (418.7598, 120.0211) -> (418.6419, 119.9686)
  line L1075 (418.6419, 119.9686) -> (418.5206, 119.9245)
  line L1076 (418.5206, 119.9245) -> (418.3965, 119.8889)
  line L1077 (418.3965, 119.8889) -> (418.2703, 119.8621)
  line L1078 (418.2703, 119.8621) -> (418.1425, 119.8441)
  line L1079 (418.1425, 119.8441) -> (418.0137, 119.8351)
  line L1080 (418.0137, 119.8351) -> (417.8846, 119.8351)
  line L1081 (417.8846, 119.8351) -> (417.7559, 119.8441)
  line L1082 (417.7559, 119.8441) -> (417.6281, 119.8621)
  line L1083 (417.6281, 119.8621) -> (417.5018, 119.8889)
  line L1084 (417.5018, 119.8889) -> (417.3778, 119.9245)
  line L1085 (417.3778, 119.9245) -> (417.2565, 119.9686)
  line L1086 (417.2565, 119.9686) -> (417.1386, 120.0211)
  line L1087 (417.1386, 120.0211) -> (417.0246, 120.0817)
  line L1088 (417.0246, 120.0817) -> (416.9152, 120.1501)
  line L1089 (416.9152, 120.1501) -> (416.8107, 120.226)
  line L1090 (416.8107, 120.226) -> (416.7119, 120.3089)
  line L1091 (416.7119, 120.3089) -> (416.619, 120.3986)
  line L1092 (416.619, 120.3986) -> (416.5327, 120.4945)
  line L1093 (416.5327, 120.4945) -> (416.4532, 120.5962)
  line L1094 (416.4532, 120.5962) -> (416.381, 120.7032)
  line L1095 (416.381, 120.7032) -> (416.3165, 120.815)
  line L1096 (416.3165, 120.815) -> (416.2599, 120.931)
  line L1097 (416.2599, 120.931) -> (416.2116, 121.0507)
  line L1098 (416.2116, 121.0507) -> (416.1717, 121.1734)
  line L1099 (416.1717, 121.1734) -> (416.1405, 121.2986)
  line L1100 (416.1405, 121.2986) -> (416.1181, 121.4258)
  line L1101 (416.1181, 121.4258) -> (416.1046, 121.5541)
  line L1102 (416.1046, 121.5541) -> (416.1001, 121.6831)
  line L1103 (416.1001, 121.6831) -> (416.1046, 121.8121)
  line L1104 (416.1046, 121.8121) -> (416.1181, 121.9404)
  line L1105 (416.1181, 121.9404) -> (416.1405, 122.0676)
  line L1106 (416.1405, 122.0676) -> (416.1717, 122.1928)
  line L1107 (416.1717, 122.1928) -> (416.2116, 122.3155)
  line L1108 (416.2116, 122.3155) -> (416.2599, 122.4352)
  line L1109 (416.2599, 122.4352) -> (416.3165, 122.5512)
  line L1110 (416.3165, 122.5512) -> (416.381, 122.663)
  line L1111 (416.381, 122.663) -> (416.4532, 122.77)
  line L1112 (416.4532, 122.77) -> (416.5327, 122.8717)
  line L1113 (416.5327, 122.8717) -> (416.619, 122.9676)
  line L1114 (416.619, 122.9676) -> (416.7119, 123.0573)
  line L1115 (416.7119, 123.0573) -> (416.8107, 123.1402)
  line L1116 (416.8107, 123.1402) -> (416.9152, 123.2161)
  line L1117 (416.9152, 123.2161) -> (417.0246, 123.2845)
  line L1118 (417.0246, 123.2845) -> (417.1386, 123.3451)
  line L1119 (417.1386, 123.3451) -> (417.2565, 123.3976)
  line L1120 (417.2565, 123.3976) -> (417.3778, 123.4417)
  line L1121 (417.3778, 123.4417) -> (417.5018, 123.4773)
  line L1122 (417.5018, 123.4773) -> (417.6281, 123.5041)
  line L1123 (417.6281, 123.5041) -> (417.7559, 123.5221)
  line L1124 (417.7559, 123.5221) -> (417.8846, 123.5311)
  line L1125 (417.8846, 123.5311) -> (418.0137, 123.5311)
  line L1126 (418.0137, 123.5311) -> (418.1425, 123.5221)
  line L1127 (418.1425, 123.5221) -> (418.2703, 123.5041)
  line L1128 (418.2703, 123.5041) -> (418.3965, 123.4773)
  line L1129 (418.3965, 123.4773) -> (418.5206, 123.4417)
  line L1130 (418.5206, 123.4417) -> (418.6419, 123.3976)
  line L1131 (418.6419, 123.3976) -> (418.7598, 123.3451)
  line L1132 (418.7598, 123.3451) -> (418.8737, 123.2845)
  line L1133 (418.8737, 123.2845) -> (418.9832, 123.2161)
  line L1134 (418.9832, 123.2161) -> (419.0876, 123.1402)
  line L1135 (419.0876, 123.1402) -> (419.1865, 123.0573)
  line L1136 (419.1865, 123.0573) -> (419.2793, 122.9676)
  line L1137 (419.2793, 122.9676) -> (419.3657, 122.8717)
  line L1138 (419.3657, 122.8717) -> (419.4451, 122.77)
  line L1139 (419.4451, 122.77) -> (419.5173, 122.663)
  line L1140 (419.5173, 122.663) -> (419.5819, 122.5512)
  line L1141 (419.5819, 122.5512) -> (419.6384, 122.4352)
  line L1142 (419.6384, 122.4352) -> (419.6868, 122.3155)
  line L1143 (419.6868, 122.3155) -> (419.7267, 122.1928)
  line L1144 (419.7267, 122.1928) -> (419.7579, 122.0676)
  line L1145 (419.7579, 122.0676) -> (419.7803, 121.9404)
  line L1146 (419.7803, 121.9404) -> (419.7938, 121.8121)
  line L1147 (419.7938, 121.8121) -> (419.7983, 121.6831)
  line L1148 (274.4343, 93.4397) -> (418.432, 93.4397)
  line L1149 (418.432, 93.4397) -> (418.432, 13.1401)
  line L1150 (418.432, 13.1401) -> (274.4343, 13.1401)
  line L1151 (274.4343, 13.1401) -> (274.4343, 93.4397)
  line L1152 (274.3835, 93.4473) -> (418.4269, 93.4473)
  line L1153 (418.4269, 93.4473) -> (418.4269, 13.1426)
  line L1154 (418.4269, 13.1426) -> (274.4064, 13.1426)
  line L1155 (274.4064, 13.1426) -> (274.2692, 93.4092)
  line L1156 (327.0656, 36.4675) -> (327.1063, 37.3692)
  line L1157 (327.1063, 37.3692) -> (327.2384, 38.2658)
  line L1158 (327.2384, 38.2658) -> (327.4492, 39.1446)
  line L1159 (327.4492, 39.1446) -> (327.7464, 40.0031)
  line L1160 (327.7464, 40.0031) -> (328.1223, 40.8236)
  line L1161 (328.1223, 40.8236) -> (328.5744, 41.611)
  line L1162 (328.5744, 41.611) -> (329.1002, 42.3476)
  line L1163 (329.1002, 42.3476) -> (329.692, 43.0334)
  line L1164 (329.692, 43.0334) -> (330.3499, 43.6557)
  line L1165 (330.3499, 43.6557) -> (331.0611, 44.2145)
  line L1166 (331.0611, 44.2145) -> (331.8231, 44.7047)
  line L1167 (331.8231, 44.7047) -> (332.6282, 45.1212)
  line L1168 (332.6282, 45.1212) -> (333.469, 45.4565)
  line L1169 (333.469, 45.4565) -> (334.3351, 45.7131)
  line L1170 (334.3351, 45.7131) -> (335.2241, 45.8832)
  line L1171 (335.2241, 45.8832) -> (336.1284, 45.9671)
  line L1172 (336.1284, 45.9671) -> (337.0301, 45.9671)
  line L1173 (337.0301, 45.9671) -> (337.9343, 45.8832)
  line L1174 (337.9343, 45.8832) -> (338.8233, 45.7131)
  line L1175 (338.8233, 45.7131) -> (339.692, 45.4565)
  line L1176 (339.692, 45.4565) -> (340.5302, 45.1212)
  line L1177 (340.5302, 45.1212) -> (341.3379, 44.7047)
  line L1178 (341.3379, 44.7047) -> (342.0974, 44.2145)
  line L1179 (342.0974, 44.2145) -> (342.8086, 43.6557)
  line L1180 (342.8086, 43.6557) -> (343.4664, 43.0334)
  line L1181 (343.4664, 43.0334) -> (344.0582, 42.3476)
  line L1182 (344.0582, 42.3476) -> (344.584, 41.611)
  line L1183 (344.584, 41.611) -> (345.0361, 40.8236)
  line L1184 (345.0361, 40.8236) -> (345.4121, 40.0031)
  line L1185 (345.4121, 40.0031) -> (345.7092, 39.1446)
  line L1186 (345.7092, 39.1446) -> (345.9201, 38.2658)
  line L1187 (345.9201, 38.2658) -> (346.0521, 37.3692)
  line L1188 (346.0521, 37.3692) -> (346.0928, 36.4675)
  line L1189 (346.0928, 36.4675) -> (346.0521, 35.5607)
  line L1190 (346.0521, 35.5607) -> (345.9201, 34.6641)
  line L1191 (345.9201, 34.6641) -> (345.7092, 33.7852)
  line L1192 (345.7092, 33.7852) -> (345.4121, 32.9292)
  line L1193 (345.4121, 32.9292) -> (345.0361, 32.1063)
  line L1194 (345.0361, 32.1063) -> (344.584, 31.3214)
  line L1195 (344.584, 31.3214) -> (344.0582, 30.5823)
  line L1196 (344.0582, 30.5823) -> (343.4664, 29.899)
  line L1197 (343.4664, 29.899) -> (342.8086, 29.2742)
  line L1198 (342.8086, 29.2742) -> (342.0974, 28.7154)
  line L1199 (342.0974, 28.7154) -> (341.3379, 28.2252)
  line L1200 (341.3379, 28.2252) -> (340.5302, 27.8111)
  line L1201 (340.5302, 27.8111) -> (339.692, 27.4759)
  line L1202 (339.692, 27.4759) -> (338.8233, 27.2219)
  line L1203 (338.8233, 27.2219) -> (337.9343, 27.0491)
  line L1204 (337.9343, 27.0491) -> (337.0301, 26.9628)
  line L1205 (337.0301, 26.9628) -> (336.1284, 26.9628)
  line L1206 (336.1284, 26.9628) -> (335.2241, 27.0491)
  line L1207 (335.2241, 27.0491) -> (334.3351, 27.2219)
  line L1208 (334.3351, 27.2219) -> (333.469, 27.4759)
  line L1209 (333.469, 27.4759) -> (332.6282, 27.8111)
  line L1210 (332.6282, 27.8111) -> (331.8231, 28.2252)
  line L1211 (331.8231, 28.2252) -> (331.0611, 28.7154)
  line L1212 (331.0611, 28.7154) -> (330.3499, 29.2742)
  line L1213 (330.3499, 29.2742) -> (329.692, 29.899)
  line L1214 (329.692, 29.899) -> (329.1002, 30.5823)
  line L1215 (329.1002, 30.5823) -> (328.5744, 31.3214)
  line L1216 (328.5744, 31.3214) -> (328.1223, 32.1063)
  line L1217 (328.1223, 32.1063) -> (327.7464, 32.9292)
  line L1218 (327.7464, 32.9292) -> (327.4492, 33.7852)
  line L1219 (327.4492, 33.7852) -> (327.2384, 34.6641)
  line L1220 (327.2384, 34.6641) -> (327.1063, 35.5607)
  line L1221 (327.1063, 35.5607) -> (327.0656, 36.4675)
  line L1222 (288.7523, 36.4675) -> (288.7955, 37.3692)
  line L1223 (288.7955, 37.3692) -> (288.925, 38.2658)
  line L1224 (288.925, 38.2658) -> (289.1384, 39.1446)
  line L1225 (289.1384, 39.1446) -> (289.433, 40.0031)
  line L1226 (289.433, 40.0031) -> (289.8115, 40.8236)
  line L1227 (289.8115, 40.8236) -> (290.2636, 41.611)
  line L1228 (290.2636, 41.611) -> (290.7894, 42.3476)
  line L1229 (290.7894, 42.3476) -> (291.3812, 43.0334)
  line L1230 (291.3812, 43.0334) -> (292.0365, 43.6557)
  line L1231 (292.0365, 43.6557) -> (292.7477, 44.2145)
  line L1232 (292.7477, 44.2145) -> (293.5097, 44.7047)
  line L1233 (293.5097, 44.7047) -> (294.3123, 45.1212)
  line L1234 (294.3123, 45.1212) -> (295.1556, 45.4565)
  line L1235 (295.1556, 45.4565) -> (296.0243, 45.7131)
  line L1236 (296.0243, 45.7131) -> (296.9133, 45.8832)
  line L1237 (296.9133, 45.8832) -> (297.8125, 45.9671)
  line L1238 (297.8125, 45.9671) -> (298.7192, 45.9671)
  line L1239 (298.7192, 45.9671) -> (299.6235, 45.8832)
  line L1240 (299.6235, 45.8832) -> (300.5125, 45.7131)
  line L1241 (300.5125, 45.7131) -> (301.3786, 45.4565)
  line L1242 (301.3786, 45.4565) -> (302.2194, 45.1212)
  line L1243 (302.2194, 45.1212) -> (303.022, 44.7047)
  line L1244 (303.022, 44.7047) -> (303.784, 44.2145)
  line L1245 (303.784, 44.2145) -> (304.4977, 43.6557)
  line L1246 (304.4977, 43.6557) -> (305.1531, 43.0334)
  line L1247 (305.1531, 43.0334) -> (305.7474, 42.3476)
  line L1248 (305.7474, 42.3476) -> (306.2732, 41.611)
  line L1249 (306.2732, 41.611) -> (306.7228, 40.8236)
  line L1250 (306.7228, 40.8236) -> (307.1012, 40.0031)
  line L1251 (307.1012, 40.0031) -> (307.3984, 39.1446)
  line L1252 (307.3984, 39.1446) -> (307.6092, 38.2658)
  line L1253 (307.6092, 38.2658) -> (307.7388, 37.3692)
  line L1254 (307.7388, 37.3692) -> (307.782, 36.4675)
  line L1255 (307.782, 36.4675) -> (307.7388, 35.5607)
  line L1256 (307.7388, 35.5607) -> (307.6092, 34.6641)
  line L1257 (307.6092, 34.6641) -> (307.3984, 33.7852)
  line L1258 (307.3984, 33.7852) -> (307.1012, 32.9292)
  line L1259 (307.1012, 32.9292) -> (306.7228, 32.1063)
  line L1260 (306.7228, 32.1063) -> (306.2732, 31.3214)
  line L1261 (306.2732, 31.3214) -> (305.7474, 30.5823)
  line L1262 (305.7474, 30.5823) -> (305.1531, 29.899)
  line L1263 (305.1531, 29.899) -> (304.4977, 29.2742)
  line L1264 (304.4977, 29.2742) -> (303.784, 28.7154)
  line L1265 (303.784, 28.7154) -> (303.022, 28.2252)
  line L1266 (303.022, 28.2252) -> (302.2194, 27.8111)
  line L1267 (302.2194, 27.8111) -> (301.3786, 27.4759)
  line L1268 (301.3786, 27.4759) -> (300.5125, 27.2219)
  line L1269 (300.5125, 27.2219) -> (299.6235, 27.0491)
  line L1270 (299.6235, 27.0491) -> (298.7192, 26.9628)
  line L1271 (298.7192, 26.9628) -> (297.8125, 26.9628)
  line L1272 (297.8125, 26.9628) -> (296.9133, 27.0491)
  line L1273 (296.9133, 27.0491) -> (296.0243, 27.2219)
  line L1274 (296.0243, 27.2219) -> (295.1556, 27.4759)
  line L1275 (295.1556, 27.4759) -> (294.3123, 27.8111)
  line L1276 (294.3123, 27.8111) -> (293.5097, 28.2252)
  line L1277 (293.5097, 28.2252) -> (292.7477, 28.7154)
  line L1278 (292.7477, 28.7154) -> (292.0365, 29.2742)
  line L1279 (292.0365, 29.2742) -> (291.3812, 29.899)
  line L1280 (291.3812, 29.899) -> (290.7894, 30.5823)
  line L1281 (290.7894, 30.5823) -> (290.2636, 31.3214)
  line L1282 (290.2636, 31.3214) -> (289.8115, 32.1063)
  line L1283 (289.8115, 32.1063) -> (289.433, 32.9292)
  line L1284 (289.433, 32.9292) -> (289.1384, 33.7852)
  line L1285 (289.1384, 33.7852) -> (288.925, 34.6641)
  line L1286 (288.925, 34.6641) -> (288.7955, 35.5607)
  line L1287 (288.7955, 35.5607) -> (288.7523, 36.4675)
  line L1288 (280.2534, 89.1445) -> (280.2489, 89.0155)
  line L1289 (280.2489, 89.0155) -> (280.2354, 88.8872)
  line L1290 (280.2354, 88.8872) -> (280.213, 88.7601)
  line L1291 (280.213, 88.7601) -> (280.1818, 88.6348)
  line L1292 (280.1818, 88.6348) -> (280.1419, 88.5121)
  line L1293 (280.1419, 88.5121) -> (280.0936, 88.3924)
  line L1294 (280.0936, 88.3924) -> (280.037, 88.2764)
  line L1295 (280.037, 88.2764) -> (279.9725, 88.1646)
  line L1296 (279.9725, 88.1646) -> (279.9003, 88.0576)
  line L1297 (279.9003, 88.0576) -> (279.8208, 87.9559)
  line L1298 (279.8208, 87.9559) -> (279.7345, 87.86)
  line L1299 (279.7345, 87.86) -> (279.6416, 87.7704)
  line L1300 (279.6416, 87.7704) -> (279.5428, 87.6874)
  line L1301 (279.5428, 87.6874) -> (279.4383, 87.6115)
  line L1302 (279.4383, 87.6115) -> (279.3289, 87.5431)
  line L1303 (279.3289, 87.5431) -> (279.2149, 87.4825)
  line L1304 (279.2149, 87.4825) -> (279.097, 87.43)
  line L1305 (279.097, 87.43) -> (278.9757, 87.3859)